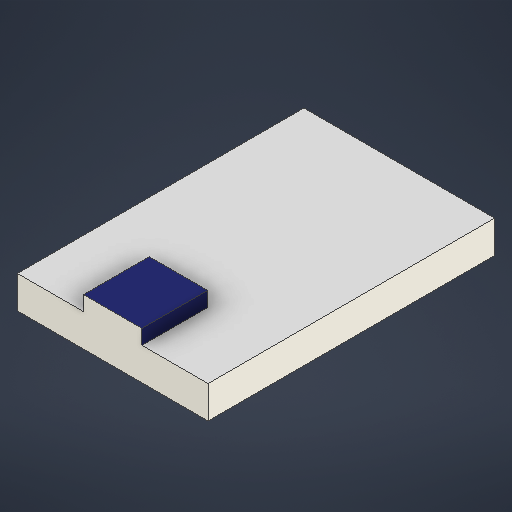
# Autodesk Inventor part: Breadboard
Saved by Autodesk Inventor 2025 (Build 290162000, 162)
## iProperties
Created: 2024-04-22
Part Number: Breadboard
Material: Generic
Document SubType Name: Modeling
Designer: conno
Density: 1 g/cm^3
Appearance: Default
BreadboardWidth: 2.177 in
BreadboardLength: 3.271 in
BreadboardHeight: 0.370 in
Author: conno
Autodesk Inventor part; units mm, degrees
ref_plane "YZ Plane" through (0, 0, 0) normal (1, 0, 0) x (0, 1, 0)
ref_plane "XZ Plane" through (0, 0, 0) normal (0, 1, 0) x (-1, 0, 0)
ref_plane "XY Plane" through (0, 0, 0) normal (0, 0, 1) x (1, 0, 0)
sketch "Sketch1" plane through (0, 0, 0) normal (0, 1, 0) x (-1, 0, 0)
  line L0 (-27.6479, 41.5354) -> (27.6479, 41.5354)
  line L1 (27.6479, 41.5354) -> (27.6479, -41.5354)
  line L2 (27.6479, -41.5354) -> (-27.6479, -41.5353)
  line L3 (-27.6479, -41.5353) -> (-27.6479, 41.5354)
  line L4 (-27.6479, 41.5354) -> (27.6479, -41.5354) construction
  line L5 (27.6479, 41.5354) -> (-27.6479, -41.5353) construction
  point P0 (0, 0)
  dimension "BreadboardWidth" = 55.2958
  dimension "BreadboardLength" = 83.0707
  constraints: 12 end point, 2 midpoint, 2 parallel, 1 horizontal, 1 perpendicular
  measures "BreadboardWidth" distance of L1.end L2.end
  measures "BreadboardLength" distance of L2.end L0.start
extrude "Breadbord" add sketch "Sketch1" along normal mid plane 9.398
sketch "Sketch2" plane through (0, 4.699, 0) normal (0, 1, 0) x (1, 0, 0)
  line L0 (8.4667, -41.5354) -> (-8.4667, -41.5354)
  line L1 (-8.4667, -41.5354) -> (-8.4667, -22.4854)
  line L2 (-8.4667, -22.4854) -> (8.4667, -22.4854)
  line L3 (8.4667, -22.4854) -> (8.4667, -41.5354)
  line L4 (8.4667, -41.5354) -> (-8.4667, -22.4854) construction
  line L5 (-8.4667, -41.5354) -> (8.4667, -22.4854) construction
  line L6 (27.6479, 41.5353) -> (-27.6479, 41.5354) projected
  line L7 (-27.6479, -41.5354) -> (27.6479, -41.5354) projected
  point P0 (0, 0)
  point P1 (0, -32.0104)
  dimension "d4" = 16.9333
  dimension "d5" = 19.05
  constraints: 12 end point, 2 midpoint, 2 parallel, 1 collinear, 1 horizontal, 1 perpendicular, 1 vertical alignment
  measures "d4" distance of L1.end L2.end
  measures "d5" distance of L0.end L1.end
extrude "LIDAR Chip" add sketch "Sketch2" along normal blind 4.2672
body "Solid1"
